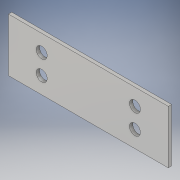
# Autodesk Inventor part: longsides
Saved by Autodesk Inventor 2017 (Build 210142000, 142)
## iProperties
Created: 2017-07-28
Part Number: longsides
Material: Generic
Document SubType Name: Modeling
Designer: Kai
Density: 1 g/cm^3
Appearance: Aluminum - Dark
Author: Kai
Autodesk Inventor part; units mm, degrees
ref_plane "YZ Plane" through (0, 0, 0) normal (1, 0, 0) x (0, 1, 0)
ref_plane "XZ Plane" through (0, 0, 0) normal (0, 1, 0) x (-1, 0, 0)
ref_plane "XY Plane" through (0, 0, 0) normal (0, 0, 1) x (1, 0, 0)
sketch "Sketch1" plane through (0, 0, 0) normal (0, 0, 1) x (1, 0, 0)
  line L0 (0, 0) -> (-304.8, 0)
  line L1 (-304.8, 0) -> (-304.8, 101.6)
  line L2 (-304.8, 101.6) -> (0, 101.6)
  line L3 (0, 101.6) -> (0, 0)
  dimension "d0" = 304.8
  dimension "d1" = 101.6
  constraints: 8 end point, 2 parallel, 1 horizontal, 1 perpendicular
  measures "d0" distance of L1.end L2.end
  measures "d1" distance of L0.end L1.end
extrude "Extrusion1" add sketch "Sketch1" along normal blind 6.35
sketch "Sketch2" plane through (0, 0, 6.35) normal (0, 0, 1) x (1, 0, 0)
  circle A0 centre (-241.3, 69.85) radius 10.5029
  line L0 (-304.8, 101.6) -> (0, 101.6) projected
  line L1 (-304.8, 101.6) -> (-304.8, 0) projected
  circle A1 centre (-241.3, 31.75) radius 10.5029
  circle A2 centre (-63.5, 69.85) radius 10.5029
  circle A3 centre (-63.5, 31.75) radius 10.5029
  point P0 (0, 0)
  dimension "d4" = 21.0058
  dimension "d5" = 31.75
  dimension "d6" = 63.5
  dimension "d9" = 38.1
  dimension "d12" = 177.8
  constraints: 4 centre point, 1 horizontal, 1 vertical, 6 other
  measures "d4" diameter of A0
  measures "d5" distance from line of L0 A0.centre
  measures "d6" distance from line of L1 A0.centre
  measures "d9" distance of A0.centre A1.centre
  measures "d12" distance of A0.centre A2.centre
extrude "Extrusion2" cut sketch "Sketch2" against normal blind 25.4
body "Solid1"
